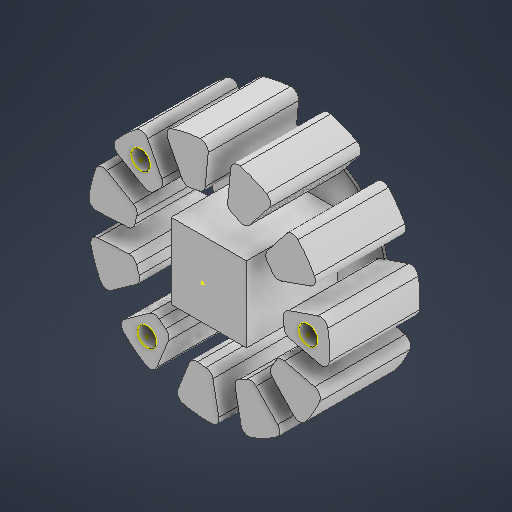
# Autodesk Inventor part: новая сиська 2
Saved by Autodesk Inventor 2025 (Build 290162000, 162)
## iProperties
Created: 2025-10-03
Part Number: новая сиська 2
Material: Типовые
Document SubType Name: Modeling
Designer: Phantom
Density: 1 g/cm^3
Appearance: По умолчанию
Author: Phantom
Autodesk Inventor part; units mm, degrees
ref_plane "YZ Plane" through (0, 0, 0) normal (1, 0, 0) x (0, 1, 0)
ref_plane "XZ Plane" through (0, 0, 0) normal (0, 1, 0) x (-1, 0, 0)
ref_plane "XY Plane" through (0, 0, 0) normal (0, 0, 1) x (1, 0, 0)
sketch "Эскиз1" plane through (0, 0, 0) normal (0, 0, 1) x (1, 0, 0)
  line L0 (14.4486, -11.4139) -> (14.4486, 13.5861)
  line L1 (14.4486, 13.5861) -> (-10.5514, 13.5861)
  line L2 (-10.5514, 13.5861) -> (-10.5514, -11.4139)
  line L3 (-10.5514, -11.4139) -> (14.4486, -11.4139)
  arc A0 (15.9584, -36.3802) -> (24.3412, -32.0586) centre (1.9486, 1.0861) ccw
  arc A1 (24.3412, -32.0586) -> (24.751, -28.2619) centre (22.9416, -29.9871) ccw
  line L4 (24.751, -28.2619) -> (17.6443, -20.8086)
  arc A2 (17.6443, -20.8086) -> (14.5647, -20.3806) centre (15.835, -22.5338) ccw
  arc A3 (12.1055, -21.6572) -> (14.5647, -20.3806) centre (1.5601, 1.663) ccw
  arc A4 (12.1055, -21.6572) -> (10.6807, -24.4083) centre (13.1356, -23.9352) ccw
  line L5 (10.6807, -24.4083) -> (12.628, -34.5117)
  arc A5 (12.628, -34.5117) -> (15.9584, -36.3802) centre (15.0828, -34.0386) ccw
  arc A6 (22.7879, -12.5396) -> (24.1684, -10.1484) centre (1.9486, 1.0861) ccw
  arc A7 (22.7879, -12.5396) -> (23.071, -15.633) centre (24.8803, -13.9078) ccw
  line L6 (23.071, -15.633) -> (30.1783, -23.0869)
  arc A8 (30.1783, -23.0869) -> (33.9902, -22.8582) centre (31.9876, -21.3617) ccw
  arc A9 (33.9902, -22.8582) -> (38.7058, -14.6906) centre (1.9486, 1.0861) ccw
  arc A10 (38.7058, -14.6906) -> (36.9979, -11.2751) centre (36.4085, -13.7046) ccw
  line L7 (36.9979, -11.2751) -> (26.9889, -8.8469)
  arc A11 (26.9889, -8.8469) -> (24.1684, -10.1484) centre (26.3995, -11.2765) ccw
  arc A12 (-6.5214, -38.0069) -> (2.867, -38.9034) centre (1.9486, 1.0861) ccw
  arc A13 (2.867, -38.9034) -> (5.2645, -35.9309) centre (2.8096, -36.404) ccw
  line L8 (5.2645, -35.9309) -> (3.3153, -25.8177)
  arc A14 (3.3153, -25.8177) -> (0.9598, -23.7928) centre (0.8605, -26.2908) ccw
  arc A15 (-1.7889, -23.5303) -> (0.9598, -23.7928) centre (1.9486, 1.0861) ccw
  arc A16 (-1.7889, -23.5303) -> (-4.4851, -25.0729) centre (-2.1641, -26.002) ccw
  line L9 (-4.4851, -25.0729) -> (-8.3129, -34.6344)
  arc A17 (-8.3129, -34.6344) -> (-6.5214, -38.0069) centre (-5.992, -35.5636) ccw
  arc A18 (-26.3121, -27.2218) -> (-18.8987, -33.0517) centre (1.9486, 1.0861) ccw
  arc A19 (-18.8987, -33.0517) -> (-15.2748, -31.8473) centre (-17.5957, -30.9181) ccw
  line L10 (-15.2748, -31.8473) -> (-11.447, -22.2857)
  arc A20 (-11.447, -22.2857) -> (-12.3338, -19.3088) centre (-13.7679, -21.3566) ccw
  arc A21 (-14.5042, -17.602) -> (-12.3338, -19.3088) centre (1.9486, 1.0861) ccw
  arc A22 (-14.5042, -17.602) -> (-17.6063, -17.4419) centre (-16.1562, -19.4784) ccw
  line L11 (-17.6063, -17.4419) -> (-25.9959, -23.4161)
  arc A23 (-25.9959, -23.4161) -> (-26.3121, -27.2218) centre (-24.5458, -25.4526) ccw
  arc A24 (-37.1302, -7.4492) -> (-34.0456, -16.3616) centre (1.9486, 1.0861) ccw
  arc A25 (-34.0456, -16.3616) -> (-30.3458, -17.3076) centre (-31.7959, -15.2711) ccw
  line L12 (-30.3458, -17.3076) -> (-21.9562, -11.3334)
  arc A26 (-21.9562, -11.3334) -> (-21.0929, -8.3495) centre (-23.4064, -9.2969) ccw
  arc A27 (-21.9959, -5.7403) -> (-21.0929, -8.3495) centre (1.9486, 1.0861) ccw
  arc A28 (-21.9959, -5.7403) -> (-24.5191, -3.9285) centre (-24.4001, -6.4257) ccw
  line L13 (-24.5191, -3.9285) -> (-34.8067, -4.4186)
  arc A29 (-34.8067, -4.4186) -> (-37.1302, -7.4492) centre (-34.6878, -6.9157) ccw
  circle A30 centre (-30.0197, 9.012) radius 3.1
  arc A31 (-35.5411, 15.0333) -> (-37.7646, 5.8681) centre (1.9486, 1.0861) ccw
  arc A32 (-37.7646, 5.8681) -> (-35.1636, 3.072) centre (-35.2825, 5.5692) ccw
  line L14 (-35.1636, 3.072) -> (-24.8759, 3.5621)
  arc A33 (-24.8759, 3.5621) -> (-22.5364, 5.6055) centre (-24.9949, 6.0592) ccw
  arc A34 (-21.8854, 8.2888) -> (-22.5364, 5.6055) centre (1.9486, 1.0861) ccw
  arc A35 (-21.8854, 8.2888) -> (-23.0285, 11.177) centre (-24.2785, 9.012) ccw
  line L15 (-23.0285, 11.177) -> (-31.948, 16.3267)
  arc A36 (-31.948, 16.3267) -> (-35.5411, 15.0333) centre (-33.198, 14.1616) ccw
  arc A37 (-14.2078, 20.031) -> (-16.2061, 18.1256) centre (1.9486, 1.0861) ccw
  arc A38 (-14.2078, 20.031) -> (-13.6079, 23.0788) centre (-15.83, 21.9332) ccw
  line L16 (-13.6079, 23.0788) -> (-18.3274, 32.2332)
  arc A39 (-18.3274, 32.2332) -> (-22.0493, 33.0877) centre (-20.5494, 31.0876) ccw
  arc A40 (-22.0493, 33.0877) -> (-28.8749, 26.5795) centre (1.9486, 1.0861) ccw
  arc A41 (-28.8749, 26.5795) -> (-28.1985, 22.8211) centre (-26.9485, 24.9861) ccw
  line L17 (-28.1985, 22.8211) -> (-19.279, 17.6714)
  arc A42 (-19.279, 17.6714) -> (-16.2061, 18.1256) centre (-18.029, 19.8365) ccw
  line L18 (0.7517, 27.998) -> (1.7307, 38.2507)
  arc A43 (1.7307, 38.2507) -> (-0.9384, 40.9818) centre (-0.7579, 38.4883) ccw
  arc A44 (-0.9384, 40.9818) -> (-10.1991, 39.1969) centre (1.9486, 1.0861) ccw
  arc A45 (-10.1991, 39.1969) -> (-11.6619, 35.6694) centre (-9.4398, 36.815) ccw
  line L19 (-11.6619, 35.6694) -> (-6.9425, 26.515)
  arc A46 (-6.9425, 26.515) -> (-4.1119, 25.2358) centre (-4.7204, 27.6606) ccw
  arc A47 (-1.4007, 25.7583) -> (-4.1119, 25.2358) centre (1.9486, 1.0861) ccw
  arc A48 (-1.4007, 25.7583) -> (0.7517, 27.998) centre (-1.7369, 28.2356) ccw
  arc A49 (12.4698, 23.6524) -> (9.9065, 24.6786) centre (1.9486, 1.0861) ccw
  arc A50 (12.4698, 23.6524) -> (15.4914, 24.3729) centre (13.5263, 25.9183) ccw
  line L20 (15.4914, 24.3729) -> (21.858, 32.4687)
  arc A51 (21.858, 32.4687) -> (21.0892, 36.2093) centre (19.8929, 34.0141) ccw
  arc A52 (21.0892, 36.2093) -> (12.3336, 39.7145) centre (1.9486, 1.0861) ccw
  arc A53 (12.3336, 39.7145) -> (9.1959, 37.5378) centre (11.6845, 37.3002) ccw
  line L21 (9.1959, 37.5378) -> (8.2169, 27.2852)
  arc A54 (8.2169, 27.2852) -> (9.9065, 24.6786) centre (10.7055, 27.0475) ccw
  arc A55 (36.9993, 20.5188) -> (31.4947, 28.1769) centre (1.9935, 1.1644) ccw
  arc A56 (31.4947, 28.1769) -> (27.6789, 28.0253) centre (29.6509, 26.4886) ccw
  line L22 (27.6789, 28.0253) -> (21.3482, 19.9014)
  arc A57 (21.3482, 19.9014) -> (21.3742, 16.7952) centre (23.3202, 18.3647) ccw
  arc A58 (22.9858, 14.5532) -> (21.3742, 16.7952) centre (1.9935, 1.1644) ccw
  arc A59 (22.9858, 14.5532) -> (25.9217, 13.5387) centre (25.0936, 15.8975) ccw
  line L23 (25.9217, 13.5387) -> (35.6395, 16.9503)
  arc A60 (35.6395, 16.9503) -> (36.9993, 20.5188) centre (34.8114, 19.3092) ccw
  line L24 (28.7568, -1.5592) -> (38.7658, -3.9874)
  arc A61 (38.7658, -3.9874) -> (41.849, -1.7341) centre (39.3552, -1.5579) ccw
  arc A62 (41.849, -1.7341) -> (41.4003, 7.6863) centre (1.9486, 1.0861) ccw
  arc A63 (41.4003, 7.6863) -> (38.1169, 9.6363) centre (38.9345, 7.2738) ccw
  line L25 (38.1169, 9.6363) -> (28.384, 6.2677)
  arc A64 (28.384, 6.2677) -> (26.7149, 3.648) centre (29.2017, 3.9052) ccw
  arc A65 (26.8463, 0.89) -> (26.7149, 3.648) centre (1.9486, 1.0861) ccw
  arc A66 (26.8463, 0.89) -> (28.7568, -1.5592) centre (29.3462, 0.8703) ccw
  circle A67 centre (-29.2299, -9.5296) radius 3.1
  circle A68 centre (-18.5412, -24.7008) radius 3.1
  circle A69 centre (-1.3471, -31.6848) radius 3.1
  circle A70 centre (16.8934, -28.2643) radius 3.1
  circle A71 centre (30.3889, -15.5252) radius 3.1
  circle A72 centre (34.8549, 2.4878) radius 3.1
  circle A73 centre (28.8733, 20.0558) radius 3.1
  circle A74 centre (14.3433, 31.601) radius 3.1
  circle A75 centre (-4.1219, 33.458) radius 3.1
  circle A76 centre (-20.6598, 25.0371) radius 3.1
  point P0 (0, 0)
  point P1 (0.4295, 0.4351)
  dimension "d7" = 360
  constraints: 132 point on circle, 77 centre point, 52 end point, 23 other
extrude "Выдавливание1" add sketch "Эскиз1" along normal blind 30 contours L3 L2 L1 L0 | A5 L5 A4 A3 A2 L4 A1 A0 | A6 A11 L7 A10 A9 A8 L6 A7 | A17 L9 A16 A15 A14 L8 A13 A12 | A23 L11 A22 A21 A20 L10 A19 A18 | A29 L13 A28 A27 A26 L12 A25 A24 | A30 | A36 L15 A35 A34 A33 L14 A32 A31 | A37 A42 L17 A41 A40 A39 L16 A38 | A48 A47 A46 L19 A45 A44 A43 L18 | A49 A54 L21 A53 A52 A51 L20 A50 | A60 L23 A59 A58 A57 L22 A56 A55 | A66 A65 A64 L25 A63 A62 A61 L24 | A67 | A69 | A70 | A71 | A73 | A74 | A75
sketch "Эскиз2" plane through (0, 0, 0) normal (0, 0, -1) x (-1, 0, 0)
  line L0 (-14.4486, 13.5861) -> (10.5514, 13.5861) projected
  line L1 (-14.4486, -11.4139) -> (-14.4486, 13.5861) projected
  line L2 (10.5514, -11.4139) -> (-14.4486, -11.4139) projected
  line L3 (10.5514, 13.5861) -> (10.5514, -11.4139) projected
  circle A0 centre (-1.9486, 1.0861) radius 28.7533
  point P0 (0, 0)
  constraints: 1 centre point
extrude "Выдавливание2" add sketch "Эскиз2" along normal blind 1 contours L0 L3 L2 L1 | A0
fillet "Сопряжение1" radius 2 11 edges at (-0.7846, -27.5371, 0) (15.1241, -24.4709, 0) (26.8497, -13.2906, 0) (30.6693, 2.4542, 0) (25.2752, 17.8975, 0) (12.6351, 27.7798, 0) (-3.4931, 29.3198, 0) (-17.8935, 21.8959, 0) (-25.9943, 7.8649, 0) (-25.2234, -8.3182, 0) (-15.8256, -21.5156, 0)
sketch "Эскиз3" plane through (0, 0, 30) normal (0, 0, 1) x (1, 0, 0)
  circle A0 centre (34.8549, 2.4878) radius 3.1 projected
  circle A1 centre (-20.6598, 25.0371) radius 3.1 projected
  circle A2 centre (-18.5412, -24.7008) radius 3.1 projected
  point P0 (0, 0)
